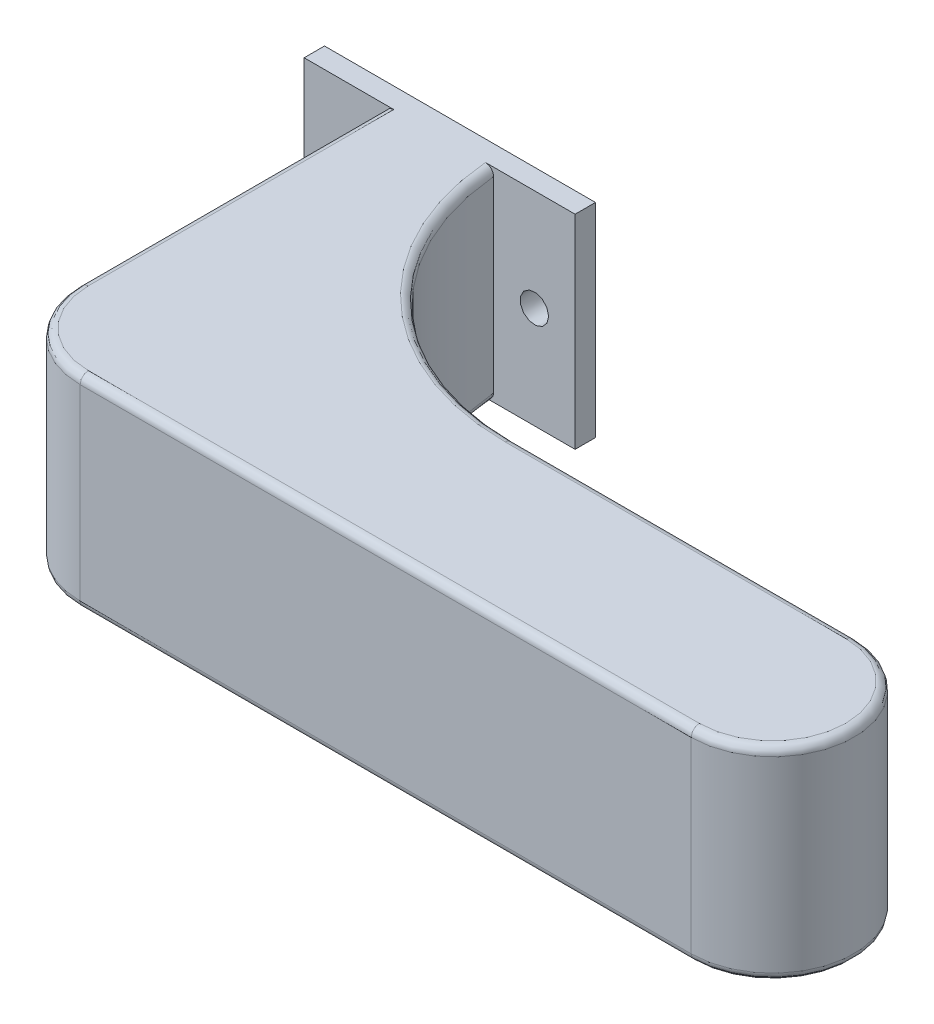
# Autodesk Inventor part: Pylon
Saved by Autodesk Inventor 2026.1 (Build 301233000, 233)
## iProperties
Created: 2025-09-15
Part Number: Pylon
Material: Generic
Document SubType Name: Modeling
Designer: mateo
Density: 1 g/cm^3
Appearance: Default
Author: mateo
Autodesk Inventor part; units mm, degrees
ref_plane "YZ Plane" through (0, 0, 0) normal (1, 0, 0) x (0, 1, 0)
ref_plane "XZ Plane" through (0, 0, 0) normal (0, 1, 0) x (-1, 0, 0)
ref_plane "XY Plane" through (0, 0, 0) normal (0, 0, 1) x (1, 0, 0)
sketch "Sketch1" plane through (0, 0, 0) normal (0, 1, 0) x (-1, 0, 0)
  line L0 (0, 0) -> (80, 0)
  line L1 (20, 5) -> (0, 5)
  line L2 (0, 5) -> (0, 0)
  line L3 (46.5184, 5) -> (46.5184, 80)
  circle A0 centre (26.5184, 80) radius 20
  line L4 (26.5184, 100) -> (-123.4816, 100)
  circle A1 centre (-123.4816, 80) radius 20
  line L5 (-123.4816, 60) -> (-39.7913, 60)
  arc A2 (20, 5) -> (-39.7913, 60) centre (-39.7913, 0) ccw
  line L6 (46.5184, 5) -> (66.5184, 5)
  line L7 (66.5184, 5) -> (66.5184, 0)
  line L8 (66.5184, 0) -> (46.5184, 0)
  point P0 (16.5184, 60)
  dimension "d1" = 75
  dimension "d2" = 40
  dimension "d3" = 150
  dimension "d4" = 140
  dimension "d7" = 40
  dimension "d10" = 5
  dimension "d11" = 5
  constraints: 18 end point, 6 point on circle, 4 horizontal, 3 centre point, 3 tangent, 2 parallel, 1 perpendicular, 1 point on line, 1 vertical
  measures "d1" distance of L3.start L3.end
  measures "d2" diameter of A0
  measures "d3" distance of L4.start L4.end
  measures "d4" distance of L5.start point (16.518, 60)
  measures "d7" diameter of A1
  measures "d10" distance of L6.end L7.end
  measures "d11" distance of L1.end L0.start
extrude "Extrusion1" add sketch "Sketch1" along normal blind 50
sketch "Sketch2" plane through (-20, 0, 5) normal (0, 0, 1) x (1, 0, 0)
  circle A0 centre (10, 25) radius 3.5
  line L0 (20, 0) -> (20, 50) projected
  line L1 (0, 50) -> (20, 50) projected
  circle A1 centre (-36.5184, 25) radius 3.5
  line L2 (-46.5184, 0) -> (-46.5184, 50) projected
  line L3 (-46.5184, 50) -> (-26.5184, 50) projected
  dimension "d14" = 7
  dimension "d15" = 10
  dimension "d16" = 25
  dimension "d17" = 7
  dimension "d18" = 10
  dimension "d22" = 25
  constraints: 2 centre point
  measures "d14" diameter of A0
  measures "d15" distance from line of L0 A0.centre
  measures "d16" distance from line of L1 A0.centre
  measures "d17" diameter of A1
  measures "d18" distance from line of A1.centre L2
  measures "d22" distance from line of A1.centre L3
extrude "Extrusion2" cut sketch "Sketch2" against normal blind 20
fillet "Fillet1" radius 2 12 edges at (-0.8289, 0, 44.1588) (143.4816, 0, 80) (48.4816, 0, 100) (-40.6606, 0, 94.1421) (-46.5184, 0, 42.5) (81.6364, 0, 60) (81.6364, 50, 60) (-0.8289, 50, 44.1588) (48.4816, 50, 100) (-40.6606, 50, 94.1421) (-46.5184, 50, 42.5) (143.4816, 50, 80)
body "Solid1"
